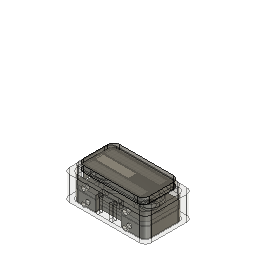
Tactile Sensor MK2 v15 (Autodesk Fusion 360 design; units mm, degrees)
Autodesk Fusion 360 part; units mm, degrees
(part 1 of 2)
sketch "Sketch1" plane through (0, 0, 0) normal (0, 0, 1) x (1, 0, 0)
  line L0 (16.51, 9.525) -> (-16.51, 9.525)
  line L1 (-16.51, 9.525) -> (-16.51, -9.525)
  line L2 (-16.51, -9.525) -> (16.51, -9.525)
  line L3 (16.51, -9.525) -> (16.51, 9.525)
  line L4 (16.51, 9.525) -> (-16.51, -9.525) construction
  line L5 (-16.51, 9.525) -> (16.51, -9.525) construction
  dimension "d1" = 33.02
  dimension "d2" = 19.05
  constraint horizontal L0
  constraint perpendicular L0 L1
  constraint parallel L0 L2
  constraint parallel L1 L3
  constraint coincident L4 origin
  constraint coincident L5 origin
  measures "d1" distance of L0.start L0.end
  measures "d2" distance of L0.start L2.end
extrude "Extrude1" add sketch "Sketch1" along normal mid plane 12.7 makes body 1
sketch "Sketch3" plane through (0, 0, 0) normal (0, 1, 0) x (1, 0, 0) in component "1"
  line L0 (21, -3) -> (-21, -3)
  line L1 (-21, -3) -> (-21, 3)
  line L2 (-21, 3) -> (21, 3)
  line L3 (21, 3) -> (21, -3)
  line L4 (21, -3) -> (-21, 3) construction
  line L5 (-21, -3) -> (21, 3) construction
  dimension "d5" = 6
  dimension "d7" = 42
  constraint horizontal L0
  constraint perpendicular L0 L1
  constraint parallel L0 L2
  constraint parallel L1 L3
  constraint coincident L4 origin
  constraint coincident L5 origin
  measures "d5" distance of L0.end L1.end
  measures "d7" distance of L1.end L2.end
extrude "Extrude1'" add sketch "Sketch3" along normal mid plane 22 separate body makes body 2 in component "1"
sketch "Sketch1 (2)" plane through (0, 0, 0) normal (0, 0, 1) x (1, 0, 0) in component "49E Hall Sensor LM393"
  line L0 (13.7, 7.8) -> (-13.7, 7.8)
  line L1 (-13.7, 7.8) -> (-13.7, -7.8)
  line L2 (-13.7, -7.8) -> (13.7, -7.8)
  line L3 (13.7, -7.8) -> (13.7, 7.8)
  line L4 (13.7, 7.8) -> (-13.7, -7.8) construction
  line L5 (-13.7, 7.8) -> (13.7, -7.8) construction
  dimension "d279" = 27.4
  dimension "d280" = 15.6
  constraint horizontal L0
  constraint perpendicular L0 L1
  constraint parallel L0 L2
  constraint parallel L1 L3
  constraint coincident L4 origin
  constraint coincident L5 origin
  measures "d279" distance of L0.start L0.end
  measures "d280" distance of L0.start L2.end
extrude "Extrude1''" add sketch "Sketch1 (2)" along normal blind 1.55 separate body makes body 3 in component "49E Hall Sensor LM393"
sketch "Sketch2" plane through (0, 0, 1.55) normal (0, 0, 1) x (-1, 0, 0) in component "49E Hall Sensor LM393"
  line L0 (-18.2, -2) -> (-14.4, -2)
  line L1 (-14.4, -2) -> (-14.4, 2)
  line L2 (-14.4, 2) -> (-18.2, 2)
  line L3 (-18.2, 2) -> (-18.2, -2)
  line L4 (-18.2, -2) -> (-14.4, 2) construction
  line L5 (-14.4, -2) -> (-18.2, 2) construction
  line L6 (-13.7, 7.8) -> (-13.7, -7.8)
  line L7 (-13.7, -7.8) -> (13.7, -7.8)
  line L8 (13.7, -7.8) -> (13.7, 7.8)
  line L9 (13.7, 7.8) -> (-13.7, 7.8)
  line L10 (0, 0) -> (-16.3, 0) construction
  line L11 (-13.7, -1.2) -> (-14.4, -1.2)
  line L12 (-14.4, -1.2) -> (-14.4, 1.2)
  line L13 (-14.4, 1.2) -> (-13.7, 1.2)
  line L14 (-13.7, 1.2) -> (-13.7, -1.2)
  line L15 (-13.7, -1.2) -> (-14.4, 1.2) construction
  line L16 (-14.4, -1.2) -> (-13.7, 1.2) construction
  point P0 (-16.3, 0)
  point P1 (-14.05, 0)
  dimension "d16" = 4
  dimension "d281" = 2.4
  dimension "d282" = 4.5
  dimension "d283" = 0.7
  constraint horizontal L0
  constraint perpendicular L0 L1
  constraint parallel L0 L2
  constraint parallel L1 L3
  constraint coincident L4 P0
  constraint coincident L5 P0
  constraint coincident L10.start origin
  constraint perpendicular L3 L10
  constraint coincident P0 L10.end
  constraint horizontal L11
  constraint perpendicular L11 L12
  constraint parallel L11 L13
  constraint parallel L12 L14
  constraint coincident L6 L11.start
  constraint coincident L15 P1
  constraint coincident L16 P1
  constraint coincident L10 P1
  constraint coincident L1 L11.end
  measures "d16" distance of L0.start L2.end
  measures "d281" distance of L11.start L13.end
  measures "d282" distance of L3 L6
  measures "d283" distance of L1 L6
extrude "Extrude2" add sketch "Sketch2" along normal blind 1 separate body contours L0 L1 L2 L3 L12 makes body 4 in component "49E Hall Sensor LM393"
extrude "Extrude4" add sketch "Sketch2" against normal blind 0.5 contours L0 L1 L2 L3 L12 | L1 L6 L11 L12 L13 L14 bodies 3 4 in component "49E Hall Sensor LM393"
sketch "Sketch7" plane through (0, 0, 3) normal (0, 0, 1) x (-1, 0, 0) in component "1"
  line L0 (21, -9) -> (-19, -9)
  line L1 (-19, -9) -> (-19, 9)
  line L2 (-19, 9) -> (21, 9)
  line L3 (21, 9) -> (21, -9)
  line L4 (21, -9) -> (-19, 9) construction
  line L5 (-19, -9) -> (21, 9) construction
  line L6 (-21, 11) -> (-21, -11)
  line L7 (-21, -11) -> (21, -11)
  line L8 (21, -11) -> (21, 11)
  line L9 (21, 11) -> (-21, 11)
  line L10 (0, 0) -> (21, 0) construction
  line L11 (19, -9) -> (19, 9)
  point P0 (1, 0)
  dimension "d301" = 2
  dimension "d302" = 2
  dimension "d455" = 2
  constraint horizontal L0
  constraint perpendicular L0 L1
  constraint parallel L0 L2
  constraint parallel L1 L3
  constraint coincident L4 P0
  constraint coincident L5 P0
  constraint coincident L10.start origin
  constraint midpoint L8 L10.end
  constraint coincident P0 L10
  constraint coincident L0.start L8
  constraint coincident L0 L11.start
  constraint coincident L2 L11.end
  constraint perpendicular L2 L11
  measures "d301" distance of L0 L7
  measures "d302" distance of L1 L6
  measures "d455" distance of L3 L11
extrude "Extrude12" cut sketch "Sketch7" against normal blind 4 contours L0 L1 L2 L11 bodies 2 in component "1"
sketch "Sketch9" plane through (0, 0, -1) normal (0, 0, 1) x (-1, 0, 0) in component "1"
  line L0 (21, -9.9472) -> (21, 9.9472)
  line L1 (-17, 9.9472) -> (-17, -9.9472) construction
  line L2 (-8, -5.8) -> (-8, 5.8) construction
  circle A0 centre (-8, -5.8) radius 0.8
  circle A1 centre (-8, 5.8) radius 0.8
  line L3 (19, 9) -> (-19, 9)
  line L4 (-19, 9) -> (-19, -9)
  line L5 (-1.5368, 0) -> (0, 0)
  line L6 (0, 0) -> (19, 0) construction
  line L7 (19, -9) -> (19, 9)
  point P0 (-1.5368, 0)
  point P1 (-8, 0)
  dimension "d53" = 11.6
  dimension "d305" = 11
  dimension "d306" = 1.6
  constraint coincident L2.start A0.centre
  constraint coincident L2.end A1.centre
  constraint equal A0 A1
  constraint coincident P0 L5.start
  constraint coincident L5.end L6.start
  constraint horizontal L5
  constraint midpoint L2 P1
  constraint coincident L6 P1
  constraint vertical L2
  constraint midpoint L6.end L7
  measures "d53" distance of L2.start L2.end
  measures "d305" distance of L2 L4
  measures "d306" diameter of A0
extrude "Extrude7" add sketch "Sketch9" along normal blind 4 bodies 2 in component "1"
sketch "Sketch15" plane through (0, 0, 3) normal (0, 0, 1) x (-1, 0, 0) in component "1"
  line L0 (-21, -11) -> (21, -11)
  line L1 (19, -9) -> (-19, -9)
  line L2 (-19, -9) -> (-19, 9)
  line L3 (-19, 9) -> (19, 9)
  line L4 (21, -11) -> (21, 11)
  line L5 (21, 11) -> (-21, 11)
  line L6 (-21, 11) -> (-21, -11)
  circle A0 centre (-8.5, 0) radius 11.5
  line L7 (0, 0) -> (-21, 0) construction
  line L8 (19, 9) -> (19, -9)
  dimension "d407" = 23
  dimension "d408" = 12.5
  constraint coincident L7.start origin
  constraint midpoint L6 L7.end
  constraint coincident A0.centre L7
  measures "d407" diameter of A0
  measures "d408" distance of L6 A0.centre
sketch "Sketch13" plane through (0, 0, -3) normal (0, 0, -1) x (1, 0, 0) in component "1"
  line L0 (21, -11) -> (21, 11)
  line L1 (21, 11) -> (-21, 11)
  line L2 (-21, 11) -> (-21, -11)
  line L3 (-21, -11) -> (21, -11)
  line L4 (-21, 6) -> (-17, 6)
  line L5 (-17, 6) -> (-17, -6)
  line L6 (-17, -6) -> (-21, -6)
  line L7 (-21, -6) -> (-21, 6)
  line L8 (-21, 6) -> (-17, -6) construction
  line L9 (-17, 6) -> (-21, -6) construction
  line L10 (0, 0) -> (-21, 0)
  point P0 (-19, 0)
  dimension "d309" = 4
  dimension "d310" = 12
  constraint horizontal L4
  constraint perpendicular L4 L5
  constraint parallel L4 L6
  constraint parallel L5 L7
  constraint coincident L2 L4.start
  constraint coincident L8 P0
  constraint coincident L9 P0
  constraint coincident L10.start origin
  constraint midpoint L7 L10.end
  constraint horizontal L10
  measures "d309" distance of L4.start L4.end
  measures "d310" distance of L4.end L5.end
sketch "Sketch3 (2)" plane through (0, 0, 0) normal (0, 1, 0) x (1, 0, 0) in component "cap 1"
  line L0 (21, -0.75) -> (-21, -0.75)
  line L1 (-21, -0.75) -> (-21, 0.75)
  line L2 (-21, 0.75) -> (21, 0.75)
  line L3 (21, 0.75) -> (21, -0.75)
  line L4 (21, -0.75) -> (-21, 0.75) construction
  line L5 (-21, -0.75) -> (21, 0.75) construction
  dimension "d5_1" = 1.5
  dimension "d7_1" = 42
  constraint horizontal L0
  constraint perpendicular L0 L1
  constraint parallel L0 L2
  constraint parallel L1 L3
  constraint coincident L4 origin
  constraint coincident L5 origin
  measures "d5_1" distance of L0.end L1.end
  measures "d7_1" distance of L1.end L2.end
extrude "Extrude1'''" add sketch "Sketch3 (2)" along normal mid plane 25 separate body makes body 5 in component "cap 1"
sketch "Sketch20" plane through (0, 0, -0.75) normal (0, 0, -1) x (1, 0, 0) in component "cap 1"
  line L0 (-21, 12.5) -> (-21, -12.5)
  line L1 (-21, -12.5) -> (21, -12.5)
  line L2 (21, -12.5) -> (21, 12.5)
  line L3 (21, 12.5) -> (-21, 12.5)
  line L4 (18.8, 10.3) -> (-21, 10.3)
  line L5 (-21, 10.3) -> (-21, -10.3)
  line L6 (-21, -10.3) -> (18.8, -10.3)
  line L7 (18.8, -10.3) -> (18.8, 10.3)
  line L8 (18.8, 10.3) -> (-21, -10.3) construction
  line L9 (-21, 10.3) -> (18.8, -10.3) construction
  line L10 (21, 0) -> (-21, 0) construction
  point P0 (-1.1, 0)
  dimension "d316" = 2.2
  dimension "d317" = 2.2
  constraint horizontal L4
  constraint perpendicular L4 L5
  constraint parallel L4 L6
  constraint parallel L5 L7
  constraint coincident L8 P0
  constraint coincident L9 P0
  constraint midpoint L2 L10.start
  constraint midpoint L0 L10.end
  constraint coincident P0 L10
  constraint coincident L0 L4.end
  measures "d316" distance of L3 L4
  measures "d317" distance of L2 L7
extrude "Extrude23" add sketch "Sketch20" along normal blind 1.5 contours L0 L4 L5 L6 L7 bodies 5 in component "cap 1"
fillet "Fillet2" radius 3.5 2 edges at (21, -12.5, 0) (21, 12.5, 0) on bodies 5 in component "cap 1"
fillet "Fillet2" radius 3.5 2 edges at (18.8, -10.3, -1.5) (18.8, 10.3, -1.5) on bodies 5 in component "cap 1"
sketch "Sketch18" plane through (0, 0, 0.75) normal (0, 0, 1) x (1, 0, 0) in component "cap 1"
  line L0 (21, -9) -> (21, 9)
  arc A0 (21, 9) -> (17.5, 12.5) centre (17.5, 9) ccw
  line L1 (17.5, 12.5) -> (-21, 12.5)
  line L2 (-21, 12.5) -> (-21, -12.5)
  line L3 (-21, -12.5) -> (17.5, -12.5)
  arc A1 (17.5, -12.5) -> (21, -9) centre (17.5, -9) ccw
  line L4 (21, -9) -> (21, 9)
  line L5 (0, 0) -> (21, 0)
  circle A2 centre (8.5, 0) radius 12.5
  constraint coincident L5.start origin
  constraint midpoint L4 L5.end
  constraint coincident L5 A2.centre
  constraint tangent L1 A2
  constraint tangent L0 A2
sketch "Sketch21" plane through (0, 0, 0.75) normal (0, 0, 1) x (-1, 0, 0) in component "cap 1"
  circle A0 centre (-8.5, 0) radius 9.5
  arc A1 (-18.8, -6.8) -> (-15.3, -10.3) centre (-15.3, -6.8) ccw
  line L0 (-18.8, -6.8) -> (-18.8, 6.8)
  arc A2 (-15.3, 10.3) -> (-18.8, 6.8) centre (-15.3, 6.8) ccw
  line L1 (-15.3, 10.3) -> (21, 10.3)
  line L2 (21, 10.3) -> (21, -10.3)
  line L3 (21, -10.3) -> (-15.3, -10.3)
  line L4 (1.8, -10.3) -> (1.8, 10.3)
  arc A3 (-21, -9) -> (-17.5, -12.5) centre (-17.5, -9) ccw
  line L5 (-17.5, -12.5) -> (21, -12.5)
  line L6 (21, -12.5) -> (21, 12.5)
  line L7 (21, 12.5) -> (-17.5, 12.5)
  arc A4 (-17.5, 12.5) -> (-21, 9) centre (-17.5, 9) ccw
  line L8 (-21, 9) -> (-21, -9)
  line L9 (0, 0) -> (-18.8, 0) construction
  dimension "d400" = 19
  dimension "d401" = 20.6
  dimension "d406" = 12.5
  constraint coincident L3 L4.start
  constraint coincident L1 L4.end
  constraint perpendicular L1 L4
  constraint coincident L9.start origin
  constraint midpoint L0 L9.end
  constraint coincident A0.centre L9
  measures "d400" diameter of A0
  measures "d401" distance of L0 L4
  measures "d406" distance of A0.centre L8
extrude "Extrude26" cut sketch "Sketch21" against normal blind 3.1 contours A0 bodies 5 in component "cap 1"
sketch "Sketch16" plane through (0, 0, 0.75) normal (0, 0, 1) x (-1, 0, 0) in component "cap 1"
  line L0 (0, 0) -> (21, 0) construction
  line L1 (-17.5, -12.5) -> (21, -12.5)
  line L2 (21, -12.5) -> (21, 12.5)
  line L3 (21, 12.5) -> (-17.5, 12.5)
  arc A0 (-21, -9) -> (-17.5, -12.5) centre (-17.5, -9) ccw
  arc A1 (-17.5, 12.5) -> (-21, 9) centre (-17.5, 9) ccw
  line L4 (-21, 9) -> (-21, -9)
  circle A2 centre (-8.5, 0) radius 9.5
  line L5 (5, -5) -> (8, -5)
  line L6 (8, -5) -> (8, 5)
  line L7 (8, 5) -> (5, 5)
  line L8 (5, 5) -> (5, -5)
  line L9 (5, -5) -> (8, 5) construction
  line L10 (8, -5) -> (5, 5) construction
  line L11 (11, -3) -> (14, -3)
  line L12 (14, -3) -> (14, 3)
  line L13 (14, 3) -> (11, 3)
  line L14 (11, 3) -> (11, -3)
  line L15 (11, -3) -> (14, 3) construction
  line L16 (14, -3) -> (11, 3) construction
  point P0 (6.5, 0)
  point P1 (12.5, 0)
  dimension "d413" = 3
  dimension "d414" = 10
  dimension "d415" = 15
  dimension "d416" = 21
  dimension "d417" = 3
  dimension "d418" = 6
  constraint coincident L0.start origin
  constraint midpoint L0.end L2
  constraint horizontal L5
  constraint perpendicular L5 L6
  constraint parallel L5 L7
  constraint parallel L6 L8
  constraint coincident L9 P0
  constraint coincident L10 P0
  constraint coincident L0 P0
  constraint horizontal L11
  constraint perpendicular L11 L12
  constraint parallel L11 L13
  constraint parallel L12 L14
  constraint coincident L15 P1
  constraint coincident L16 P1
  constraint coincident L0 P1
  measures "d413" distance of L5.start L5.end
  measures "d414" distance of L5.start L7.end
  measures "d415" distance of A2.centre P0
  measures "d416" distance of A2.centre P1
  measures "d417" distance of L11.start L11.end
  measures "d418" distance of L11.end L12.end
extrude "Extrude16" cut sketch "Sketch16" against normal blind 3.5 contours L5 L6 L7 L8 | L11 L12 L13 L14 bodies 5 in component "cap 1"
sketch "Sketch1 (3)" plane through (0, 0, 0) normal (0, 0, 1) x (1, 0, 0) in component "FSR"
  circle A0 centre (0, 0) radius 9.25
  line L0 (-8.4107, 3.85) -> (-47.4107, 3.85)
  line L1 (-47.4107, 3.85) -> (-47.4107, -3.85)
  line L2 (-47.4107, -3.85) -> (-8.4107, -3.85)
  line L3 (-8.4107, -3.85) -> (-8.4107, 3.85)
  line L4 (-8.4107, 3.85) -> (-47.4107, -3.85) construction
  line L5 (-47.4107, 3.85) -> (-8.4107, -3.85) construction
  line L6 (0, 0) -> (-43.0818, 0) construction
  point P0 (-27.9107, 0)
  point P1 (-30.0207, -4.2733)
  dimension "d244" = 18.5
  dimension "d246" = 7.7
  dimension "d247" = 39
  constraint coincident A0.centre L6.start
  constraint horizontal L0
  constraint perpendicular L0 L1
  constraint parallel L0 L2
  constraint parallel L1 L3
  constraint coincident A0 L0.start
  constraint coincident L4 P0
  constraint coincident L5 P0
  constraint coincident P0 L6
  constraint horizontal L6
  measures "d244" diameter of A0
  measures "d246" distance of L0.end L1.end
  measures "d247" distance of L1.end L2.end
extrude "Extrude1''''" add sketch "Sketch1 (3)" along normal blind 0.06 separate body makes body 6 in component "FSR"
sketch "Sketch1 (4)" plane through (0, 0, 0) normal (0, 0, -1) x (1, 0, 0) in component "termistor"
  line L0 (-2.5, 2.5) -> (18, 2.5)
  line L1 (18, 2.5) -> (18, -2.5)
  line L2 (18, -2.5) -> (-2.5, -2.5)
  line L3 (-2.5, -2.5) -> (-2.5, 2.5)
  line L4 (-2.5, 2.5) -> (18, -2.5) construction
  line L5 (18, 2.5) -> (-2.5, -2.5) construction
  line L6 (0, 0) -> (7.75, 0) construction
  line L7 (-8.4107, 3.85) -> (-47.4107, 3.85)
  line L8 (-47.4107, 3.85) -> (-47.4107, -3.85)
  line L9 (-47.4107, -3.85) -> (-8.4107, -3.85)
  arc A0 (-8.4107, -3.85) -> (-8.4107, 3.85) centre (0, 0) ccw
  point P0 (7.75, 0)
  dimension "d160" = 5
  constraint horizontal L0
  constraint perpendicular L0 L1
  constraint parallel L0 L2
  constraint parallel L1 L3
  constraint coincident L4 P0
  constraint coincident L5 P0
  constraint coincident L6.start A0.centre
  constraint horizontal L6
  constraint coincident P0 L6.end
  measures "d160" distance of L0.start L2.end
sketch "Sketch3 (3)" plane through (0, 0, 1.55) normal (0, 0, 1) x (-1, 0, 0) in component "49E Hall Sensor LM393"
  line L0 (-13.7, 7.8) -> (-13.7, 1.2)
  line L1 (-13.7, 1.2) -> (-14.4, 1.2)
  line L2 (-14.4, 1.2) -> (-14.4, -1.2)
  line L3 (-14.4, -1.2) -> (-13.7, -1.2)
  line L4 (-13.7, -1.2) -> (-13.7, -7.8)
  line L5 (-13.7, -7.8) -> (13.7, -7.8)
  line L6 (13.7, -7.8) -> (13.7, 7.8)
  line L7 (13.7, 7.8) -> (-13.7, 7.8)
  line L8 (-11.7, -7.8) -> (-11.7, 7.8)
  line L9 (0, 0) -> (-11.7, 0)
  point P0 (-11.7, -5.8)
  point P1 (-11.7, 5.8)
  dimension "d286" = 11.6
  dimension "d287" = 5.8
  dimension "d288" = 2
  constraint coincident L5 L8.start
  constraint coincident L7 L8.end
  constraint perpendicular L7 L8
  constraint coincident L8 P0
  constraint coincident L8 P1
  constraint coincident L9.start origin
  constraint midpoint L8 L9.end
  measures "d286" distance of P0 P1
  measures "d287" distance of P1 L9
  measures "d288" distance of L0 L8
hole "Hole2" at (11.7, 5.8, 1.55) at (11.7, -5.8, 1.55) direction (0, 0, -1) diameter 2 depth 2000 tip angle 118 bodies 3 in component "49E Hall Sensor LM393"
sketch "Sketch4" plane through (0, 0, 1.55) normal (0, 0, 1) x (-1, 0, 0) in component "49E Hall Sensor LM393"
  circle A0 centre (-11.7, -5.8) radius 1
  circle A1 centre (-11.7, 5.8) radius 1
  line L0 (-13.7, 7.8) -> (-13.7, 1.2)
  line L1 (-13.7, 1.2) -> (-14.4, 1.2)
  line L2 (-14.4, 1.2) -> (-14.4, -1.2)
  line L3 (-14.4, -1.2) -> (-13.7, -1.2)
  line L4 (-13.7, -1.2) -> (-13.7, -7.8)
  line L5 (-13.7, -7.8) -> (13.7, -7.8)
  line L6 (13.7, -7.8) -> (13.7, 7.8)
  line L7 (13.7, 7.8) -> (-13.7, 7.8)
  line L8 (0, 0) -> (13.7, 0)
  line L9 (11.2, -5.5) -> (16.2, -5.5)
  line L10 (16.2, -5.5) -> (16.2, 5.5)
  line L11 (16.2, 5.5) -> (11.2, 5.5)
  line L12 (11.2, 5.5) -> (11.2, -5.5)
  line L13 (11.2, -5.5) -> (16.2, 5.5) construction
  line L14 (16.2, -5.5) -> (11.2, 5.5) construction
  point P0 (13.7, 0)
  dimension "d292" = 11
  dimension "d293" = 5
  constraint coincident L8.start origin
  constraint midpoint L6 P0
  constraint horizontal L9
  constraint perpendicular L9 L10
  constraint parallel L9 L11
  constraint parallel L10 L12
  constraint coincident L13 P0
  constraint coincident L14 P0
  constraint coincident P0 L8.end
  measures "d292" distance of L9.end L10.end
  measures "d293" distance of L9.start L9.end
extrude "Extrude5" add sketch "Sketch4" along normal blind 3 contours L6 L9 L10 L11 | L6 L8 L11 L12 | L6 L8 L9 L12 bodies 3 in component "49E Hall Sensor LM393"
extrude "Extrude1'''''" add sketch "Sketch1 (4)" along normal blind 0.2 separate body contours L0 L2 L3 A0 | L0 L1 L2 A0 makes body 7 in component "termistor"
sketch "Sketch2 (2)" plane through (0, 0, 0) normal (0, 0, 1) x (-1, 0, 0) in component "termistor"
  line L0 (-18, 2.5) -> (-18, -2.5)
  line L1 (-18, -2.5) -> (2.5, -2.5)
  line L2 (2.5, -2.5) -> (2.5, 2.5)
  line L3 (2.5, 2.5) -> (-18, 2.5)
  line L4 (-18, -2.5) -> (-17.8, -2.5)
  line L5 (-17.8, -2.5) -> (-17.8, 2.5)
  line L6 (-17.8, 2.5) -> (-18, 2.5)
  line L7 (-18, 2.5) -> (-18, -2.5)
  line L8 (-18, -2.5) -> (-17.8, 2.5) construction
  line L9 (-17.8, -2.5) -> (-18, 2.5) construction
  line L10 (-18, -0.9562) -> (-17.8, -0.9562)
  line L11 (-17.8, -0.9562) -> (-17.8, 0.9562)
  line L12 (-17.8, 0.9562) -> (-18, 0.9562)
  line L13 (-18, 0.9562) -> (-18, -0.9562)
  line L14 (-18, -0.9562) -> (-17.8, 0.9562) construction
  line L15 (-17.8, -0.9562) -> (-18, 0.9562) construction
  point P0 (-17.9, 0)
  point P1 (-17.9, 0)
  dimension "d163" = 0.2
  constraint horizontal L4
  constraint perpendicular L4 L5
  constraint parallel L4 L6
  constraint parallel L5 L7
  constraint coincident L0.end L1.start
  constraint coincident L8 P1
  constraint coincident L9 P1
  constraint coincident L0.start L3.end
  constraint horizontal L10
  constraint perpendicular L10 L11
  constraint parallel L10 L12
  constraint parallel L11 L13
  constraint coincident L7 L10.start
  constraint coincident L14 P1
  constraint coincident L15 P1
  constraint coincident P1 P0
  measures "d163" distance of L5.end L0.start
extrude "Extrude2'" add sketch "Sketch2 (2)" along normal blind 7 contours L0 L3 L5 L6 L7 L12 | L0 L1 L4 L5 L7 L10 bodies 7 in component "termistor"
sketch "Sketch1 (5)" plane through (0, 0, 0) normal (0, 0, 1) x (1, 0, 0) in component "Foam"
  circle A0 centre (0, 0) radius 9.375
  dimension "d248" = 18.75
  constraint coincident A0.centre origin
  measures "d248" diameter of A0
extrude "Extrude1''''''" add sketch "Sketch1 (5)" along normal mid plane 7 separate body makes body 8 in component "Foam"
sketch "Sketch1 (6)" plane through (0, 0, 0) normal (0, 0, 1) x (1, 0, 0) in component "FSR Load plate (1)"
  circle A0 centre (0, 0) radius 11
  circle A1 centre (0, 0) radius 9
  circle A2 centre (0, 0) radius 2.65
  dimension "d257_1" = 22
  dimension "d258_1" = 18
  dimension "d388" = 5.3
  constraint coincident A0.centre A1.centre
  constraint concentric A0 A1
  measures "d257_1" diameter of A0
  measures "d258_1" diameter of A1
  measures "d388" diameter of A2
extrude "Extrude1'''''''" add sketch "Sketch1 (6)" along normal blind 6 separate body contours A1 | A2 makes body 9 in component "FSR Load plate (1)"
extrude "Extrude2''" add sketch "Sketch1 (6)" along normal blind 1 contours A0 | A1 bodies 9 in component "FSR Load plate (1)"
sketch "Sketch14" plane through (0, 0, -1) normal (0, 0, 1) x (-1, 0, 0) in component "1"
  line L0 (-19, 9) -> (-19, -9)
  line L1 (-21, 11) -> (-21, -11)
  line L2 (-21, 11) -> (21, 11)
  line L3 (21, -11) -> (-21, -11)
  circle A0 centre (-9, 0) radius 5.85 construction
  line L4 (0, 0) -> (-19, 0) construction
  circle A1 centre (-9, 0) radius 5.45
  circle A2 centre (-9, 0) radius 4.1
  line L5 (-7.4277, -11.474) -> (-7.3724, 11.4476)
  circle A3 centre (-9, 0) radius 6.6 construction
  circle A4 centre (-9, 0) radius 7
  line L6 (-19, -9) -> (19, -9)
  line L7 (19, -9) -> (19, 9)
  line L8 (19, 9) -> (-19, 9)
  circle A5 centre (-8, 5.8) radius 0.8
  circle A6 centre (-8, -5.8) radius 0.8
  dimension "d372" = 11.7
  dimension "d373" = -0.4
  dimension "d374" = -1.75
  dimension "d375" = 1.6
  dimension "d376" = 13.2
  dimension "d379" = 0.4
  dimension "d399" = 12
  constraint coincident L4.start origin
  constraint midpoint L0 L4.end
  constraint concentric A0 A3
  constraint coincident A0.centre L4
  measures "d372" diameter of A0
  measures "d375" distance of A0.centre L5
  measures "d376" diameter of A3
  measures "d399" distance of L1 A0.centre
sketch "Sketch3 (4)" plane through (0, 0, 0) normal (0, 1, 0) x (1, 0, 0) in component "cap 2"
  line L0 (21, -0.75) -> (-21, -0.75)
  line L1 (-21, -0.75) -> (-21, 0.75)
  line L2 (-21, 0.75) -> (21, 0.75)
  line L3 (21, 0.75) -> (21, -0.75)
  line L4 (21, -0.75) -> (-21, 0.75) construction
  line L5 (-21, -0.75) -> (21, 0.75) construction
  dimension "d5_1_1" = 1.5
  dimension "d7_1_1" = 42
  constraint horizontal L0
  constraint perpendicular L0 L1
  constraint parallel L0 L2
  constraint parallel L1 L3
  constraint coincident L4 origin
  constraint coincident L5 origin
  measures "d5_1_1" distance of L0.end L1.end
  measures "d7_1_1" distance of L1.end L2.end
extrude "Extrude1''''''''" add sketch "Sketch3 (4)" along normal mid plane 25 separate body makes body 10 in component "cap 2"
sketch "Sketch20 (2)" plane through (0, 0, -0.75) normal (0, 0, -1) x (1, 0, 0) in component "cap 2"
  line L0 (-21, 12.5) -> (-21, -12.5)
  line L1 (-21, -12.5) -> (21, -12.5)
  line L2 (21, -12.5) -> (21, 12.5)
  line L3 (21, 12.5) -> (-21, 12.5)
  line L4 (18.8, 10.3) -> (-21, 10.3)
  line L5 (-21, 10.3) -> (-21, -10.3)
  line L6 (-21, -10.3) -> (18.8, -10.3)
  line L7 (18.8, -10.3) -> (18.8, 10.3)
  line L8 (18.8, 10.3) -> (-21, -10.3) construction
  line L9 (-21, 10.3) -> (18.8, -10.3) construction
  line L10 (21, 0) -> (-21, 0) construction
  point P0 (-1.1, 0)
  dimension "d316_1" = 2.2
  dimension "d317_1" = 2.2
  constraint horizontal L4
  constraint perpendicular L4 L5
  constraint parallel L4 L6
  constraint parallel L5 L7
  constraint coincident L8 P0
  constraint coincident L9 P0
  constraint midpoint L2 L10.start
  constraint midpoint L0 L10.end
  constraint coincident P0 L10
  constraint coincident L0 L4.end
  measures "d316_1" distance of L3 L4
  measures "d317_1" distance of L2 L7
extrude "Extrude23'" add sketch "Sketch20 (2)" along normal blind 1.5 contours L0 L4 L5 L6 L7 bodies 10 in component "cap 2"
fillet "Fillet2'" radius 3.5 2 edges at (21, -12.5, 0) (21, 12.5, 0) on bodies 10 in component "cap 2"
fillet "Fillet2'" radius 3.5 2 edges at (18.8, -10.3, -1.5) (18.8, 10.3, -1.5) on bodies 10 in component "cap 2"
sketch "Sketch18 (2)" plane through (0, 0, 0.75) normal (0, 0, 1) x (1, 0, 0) in component "cap 2"
  line L0 (21, -9) -> (21, 9)
  arc A0 (21, 9) -> (17.5, 12.5) centre (17.5, 9) ccw
  line L1 (17.5, 12.5) -> (-21, 12.5)
  line L2 (-21, 12.5) -> (-21, -12.5)
  line L3 (-21, -12.5) -> (17.5, -12.5)
  arc A1 (17.5, -12.5) -> (21, -9) centre (17.5, -9) ccw
  line L4 (21, -9) -> (21, 9)
  line L5 (0, 0) -> (21, 0)
  circle A2 centre (8.5, 0) radius 12.5
  constraint coincident L5.start origin
  constraint midpoint L4 L5.end
  constraint coincident L5 A2.centre
  constraint tangent L1 A2
  constraint tangent L0 A2
extrude "Extrude24" add sketch "Sketch18 (2)" along normal blind 1.7 contours A2 bodies 10 in component "cap 2"
sketch "Sketch21 (2)" plane through (0, 0, 2.45) normal (0, 0, 1) x (-1, 0, 0) in component "cap 2"
  circle A0 centre (-8.5, 0) radius 12.5
  circle A1 centre (-8.5, 0) radius 11
  circle A2 centre (-8.5, 0) radius 9.25
  circle A3 centre (-8.5, 0) radius 10.5
  dimension "d327_1" = -1.5
  dimension "d328_1" = 18.5
  dimension "d329_1" = 21
  constraint concentric A0 A2
  constraint concentric A2 A3
  measures "d328_1" diameter of A2
  measures "d329_1" diameter of A3
sketch "Sketch22" plane through (0, 0, -2.25) normal (0, 0, -1) x (1, 0, 0) in component "cap 2"
  arc A0 (15.3, -10.3) -> (18.8, -6.8) centre (15.3, -6.8) ccw
  line L0 (18.8, -6.8) -> (18.8, 6.8)
  arc A1 (18.8, 6.8) -> (15.3, 10.3) centre (15.3, 6.8) ccw
  line L1 (15.3, 10.3) -> (-21, 10.3)
  line L2 (-21, 10.3) -> (-21, -10.3)
  line L3 (-21, -10.3) -> (15.3, -10.3)
  line L4 (1.8, 10.3) -> (1.8, -10.3)
  dimension "d344_1" = 17
  constraint coincident L1 L4.start
  constraint coincident L3 L4.end
  constraint perpendicular L3 L4
  measures "d344_1" distance of L0 L4
sketch "Sketch1 (7)" plane through (0, 0, 0) normal (0, 0, 1) x (1, 0, 0) in component "FSR (1)"
  circle A0 centre (0, 0) radius 9.25
  line L0 (-8.4107, 3.85) -> (-47.4107, 3.85)
  line L1 (-47.4107, 3.85) -> (-47.4107, -3.85)
  line L2 (-47.4107, -3.85) -> (-8.4107, -3.85)
  line L3 (-8.4107, -3.85) -> (-8.4107, 3.85)
  line L4 (-8.4107, 3.85) -> (-47.4107, -3.85) construction
  line L5 (-47.4107, 3.85) -> (-8.4107, -3.85) construction
  line L6 (0, 0) -> (-43.0818, 0) construction
  point P0 (-27.9107, 0)
  point P1 (-30.0207, -4.2733)
  dimension "d244_1" = 18.5
  dimension "d246_1" = 7.7
  dimension "d247_1" = 39
  constraint coincident A0.centre L6.start
  constraint horizontal L0
  constraint perpendicular L0 L1
  constraint parallel L0 L2
  constraint parallel L1 L3
  constraint coincident A0 L0.start
  constraint coincident L4 P0
  constraint coincident L5 P0
  constraint coincident P0 L6
  constraint horizontal L6
  measures "d244_1" diameter of A0
  measures "d246_1" distance of L0.end L1.end
  measures "d247_1" distance of L1.end L2.end
extrude "Extrude1'''''''''" add sketch "Sketch1 (7)" along normal blind 0.06 separate body makes body 11 in component "FSR (1)"
sketch "Sketch1 (8)" plane through (0, 0, 0) normal (0, 0, -1) x (1, 0, 0) in component "termistor (1)"
  line L0 (-2.5, 2.5) -> (18, 2.5)
  line L1 (18, 2.5) -> (18, -2.5)
  line L2 (18, -2.5) -> (-2.5, -2.5)
  line L3 (-2.5, -2.5) -> (-2.5, 2.5)
  line L4 (-2.5, 2.5) -> (18, -2.5) construction
  line L5 (18, 2.5) -> (-2.5, -2.5) construction
  line L6 (0, 0) -> (7.75, 0) construction
  line L7 (-8.4107, 3.85) -> (-47.4107, 3.85)
  line L8 (-47.4107, 3.85) -> (-47.4107, -3.85)
  line L9 (-47.4107, -3.85) -> (-8.4107, -3.85)
  arc A0 (-8.4107, -3.85) -> (-8.4107, 3.85) centre (0, 0) ccw
  point P0 (7.75, 0)
  dimension "d160_1" = 5
  constraint horizontal L0
  constraint perpendicular L0 L1
  constraint parallel L0 L2
  constraint parallel L1 L3
  constraint coincident L4 P0
  constraint coincident L5 P0
  constraint coincident L6.start A0.centre
  constraint horizontal L6
  constraint coincident P0 L6.end
  measures "d160_1" distance of L0.start L2.end
extrude "Extrude1''''''''''" add sketch "Sketch1 (8)" along normal blind 0.2 separate body contours L0 L2 L3 A0 | L0 L1 L2 A0 makes body 12 in component "termistor (1)"
sketch "Sketch2 (3)" plane through (0, 0, 0) normal (0, 0, 1) x (-1, 0, 0) in component "termistor (1)"
  line L0 (-18, 2.5) -> (-18, -2.5)
  line L1 (-18, -2.5) -> (2.5, -2.5)
  line L2 (2.5, -2.5) -> (2.5, 2.5)
  line L3 (2.5, 2.5) -> (-18, 2.5)
  line L4 (-18, -2.5) -> (-17.8, -2.5)
  line L5 (-17.8, -2.5) -> (-17.8, 2.5)
  line L6 (-17.8, 2.5) -> (-18, 2.5)
  line L7 (-18, 2.5) -> (-18, -2.5)
  line L8 (-18, -2.5) -> (-17.8, 2.5) construction
  line L9 (-17.8, -2.5) -> (-18, 2.5) construction
  line L10 (-18, -0.9562) -> (-17.8, -0.9562)
  line L11 (-17.8, -0.9562) -> (-17.8, 0.9562)
  line L12 (-17.8, 0.9562) -> (-18, 0.9562)
  line L13 (-18, 0.9562) -> (-18, -0.9562)
  line L14 (-18, -0.9562) -> (-17.8, 0.9562) construction
  line L15 (-17.8, -0.9562) -> (-18, 0.9562) construction
  point P0 (-17.9, 0)
  point P1 (-17.9, 0)
  dimension "d163_1" = 0.2
  constraint horizontal L4
  constraint perpendicular L4 L5
  constraint parallel L4 L6
  constraint parallel L5 L7
  constraint coincident L0.end L1.start
  constraint coincident L8 P1
  constraint coincident L9 P1
  constraint coincident L0.start L3.end
  constraint horizontal L10
  constraint perpendicular L10 L11
  constraint parallel L10 L12
  constraint parallel L11 L13
  constraint coincident L7 L10.start
  constraint coincident L14 P1
  constraint coincident L15 P1
  constraint coincident P1 P0
  measures "d163_1" distance of L5.end L0.start
extrude "Extrude2'''" add sketch "Sketch2 (3)" along normal blind 7 contours L0 L3 L5 L6 L7 L12 | L0 L1 L4 L5 L7 L10 bodies 12 in component "termistor (1)"
sketch "Sketch1 (9)" plane through (0, 0, 0) normal (0, 0, 1) x (1, 0, 0) in component "Foam (1)"
  circle A0 centre (0, 0) radius 9.375
  dimension "d248_1" = 18.75
  constraint coincident A0.centre origin
  measures "d248_1" diameter of A0
extrude "Extrude1'''''''''''" add sketch "Sketch1 (9)" along normal mid plane 7 separate body makes body 13 in component "Foam (1)"
sketch "Sketch27" plane through (0, 0, -2.25) normal (0, 0, -1) x (1, 0, 0) in component "cap 1"
  line L0 (-18.4, -2.523) -> (-18.4, -0.673)
  line L1 (-18.4, -0.673) -> (-17.4, -0.673)
  line L2 (-17.4, -0.673) -> (-17.4, -2.523)
  line L3 (-17.4, -2.523) -> (-18.4, -2.523)
  line L4 (-17.4, 0.673) -> (-18.4, 0.673)
  line L5 (-18.4, 0.673) -> (-18.4, 2.523)
  line L6 (-18.4, 2.523) -> (-17.4, 2.523)
  line L7 (-17.4, 2.523) -> (-17.4, 0.673)
  line L8 (-18.4, -2.85) -> (-17.4, -2.85)
  line L9 (-17.4, -2.85) -> (-17.4, -8.15)
  line L10 (-17.4, -8.15) -> (-18.4, -8.15)
  line L11 (-18.4, -8.15) -> (-18.4, -2.85)
  line L12 (-18.4, 8.15) -> (-17.4, 8.15)
  line L13 (-17.4, 8.15) -> (-17.4, 2.85)
  line L14 (-17.4, 2.85) -> (-18.4, 2.85)
  line L15 (-18.4, 2.85) -> (-18.4, 8.15)
  circle A0 centre (8.5, 0) radius 9.5
  arc A1 (15.3, -10.3) -> (18.8, -6.8) centre (15.3, -6.8) ccw
  line L16 (18.8, -6.8) -> (18.8, 6.8)
  arc A2 (18.8, 6.8) -> (15.3, 10.3) centre (15.3, 6.8) ccw
  line L17 (15.3, 10.3) -> (-21, 10.3)
  line L18 (-21, 10.3) -> (-21, -10.3)
  line L19 (-21, -10.3) -> (15.3, -10.3)
  circle A3 centre (8.5, 0) radius 11.5
  circle A4 centre (8.5, 0) radius 9.5
  arc A5 (15.3, -10.3) -> (18.8, -6.8) centre (15.3, -6.8) ccw
  line L20 (18.8, -6.8) -> (18.8, 6.8)
  arc A6 (18.8, 6.8) -> (15.3, 10.3) centre (15.3, 6.8) ccw
  line L21 (15.3, 10.3) -> (-21, 10.3)
  line L22 (-21, 10.3) -> (-21, -10.3)
  line L23 (-21, -10.3) -> (15.3, -10.3)
  line L24 (-5, -5) -> (-8, -5)
  line L25 (-8, -5) -> (-8, 5)
  line L26 (-8, 5) -> (-5, 5)
  line L27 (-5, 5) -> (-5, -5)
  line L28 (-11, -3) -> (-14, -3)
  line L29 (-14, -3) -> (-14, 3)
  line L30 (-14, 3) -> (-11, 3)
  line L31 (-11, 3) -> (-11, -3)
  dimension "d403" = 23
  constraint concentric A0 A3
  measures "d403" diameter of A3
extrude "Extrude31" cut sketch "Sketch27" against normal blind 2 contours L19 A3 L23 | L16 L17 L19 A3 L20 L21 L23 | L16 A3 L20 | L17 A3 L21 bodies 5 in component "cap 1"
extrude "Extrude3" cut sketch "Sketch1 (6)" along normal blind 3 contours A2 bodies 9 in component "FSR Load plate (1)"
sketch "Sketch16 (2)" plane through (-21, 0, 0) normal (-1, 0, 0) x (0, -1, 0) in component "1"
  circle A0 centre (9.2616, 2) radius 2.5
  line L0 (-11, 2) -> (11, 2) construction
  circle A1 centre (-6, 2) radius 2.5
  line L1 (11, -3) -> (11, 3)
  line L2 (-11, -3) -> (-11, 3)
  line L3 (11, -3) -> (-11, -3)
  dimension "d419" = 5
  dimension "d429" = 5
  dimension "d430" = 5
  constraint coincident L0 A1.centre
  constraint equal A0 A1
  constraint coincident A0.centre L0
  constraint coincident L0.end L1
  constraint horizontal L0
  constraint coincident L0.start L2
  measures "d419" diameter of A1
  measures "d429" distance of A1.centre L3
  measures "d430" distance of A1.centre L2
sketch "Sketch17" plane through (0, 0, 3) normal (0, 0, 1) x (-1, 0, 0) in component "1"
  line L0 (21, 11) -> (-21, 11)
  line L1 (-21, 11) -> (-21, -11)
  line L2 (-21, -11) -> (21, -11)
  line L3 (-19, -9) -> (-19, 9)
  line L4 (19, 9) -> (19, -9)
  line L5 (19, -9) -> (-19, -9)
  line L6 (-19, 9) -> (19, 9)
  line L7 (21, -11) -> (21, 11)
  point P0 (1, -10.5)
  point P1 (1, 10.5)
sketch "Sketch17 (2)" plane through (0, 0, 0) normal (0, 0, 1) x (1, 0, 0) in component "gen 2"
  line L0 (19, 10.5) -> (-19, 10.5)
  line L1 (-19, 10.5) -> (-19, -10.5)
  line L2 (-19, -10.5) -> (19, -10.5)
  line L3 (19, -10.5) -> (19, 10.5)
  line L4 (19, 10.5) -> (-19, -10.5) construction
  line L5 (-19, 10.5) -> (19, -10.5) construction
  line L6 (-21.25, -12.75) -> (21.25, -12.75)
  line L7 (21.25, -12.75) -> (21.25, 12.75)
  line L8 (21.25, 12.75) -> (-21.25, 12.75)
  line L9 (-21.25, 12.75) -> (-21.25, -12.75)
  line L10 (-23, -14.5) -> (23, -14.5)
  line L11 (23, -14.5) -> (23, 14.5)
  line L12 (23, 14.5) -> (-23, 14.5)
  line L13 (-23, 14.5) -> (-23, -14.5)
  dimension "d1_1_1" = 38
  dimension "d2_1_1" = 21
  dimension "d3_1_1" = 2.25
  dimension "d24_1" = 4
  constraint horizontal L0
  constraint perpendicular L0 L1
  constraint parallel L0 L2
  constraint parallel L1 L3
  constraint coincident L4 origin
  constraint coincident L5 origin
  measures "d1_1_1" distance of L0.start L0.end
  measures "d2_1_1" distance of L0.start L2.end
extrude "Extrude17" add sketch "Sketch17 (2)" against normal blind 2 separate body contours L10 L11 L12 L13 makes body 14 in component "gen 2"
extrude "Extrude18" add sketch "Sketch17 (2)" along normal blind 2 contours L6 L7 L8 L9 | L10 L11 L12 L13 bodies 14 in component "gen 2"
fillet "Fillet12" radius 3.5 6 edges at (19, 10.5, 1) (21.25, 12.75, -1) (19, -10.5, 1) (21.25, -12.75, -1) (-19, -10.5, 1) (-19, 10.5, 1) on bodies 14 in component "gen 2"
sketch "Sketch3 (5)" plane through (0, 0, 0) normal (0, 1, 0) x (1, 0, 0) in component "3"
  line L0 (21, -3) -> (-21, -3)
  line L1 (-21, -3) -> (-21, 3)
  line L2 (-21, 3) -> (21, 3)
  line L3 (21, 3) -> (21, -3)
  line L4 (21, -3) -> (-21, 3) construction
  line L5 (-21, -3) -> (21, 3) construction
  dimension "d5_1_2_2" = 6
  dimension "d7_1_2_2" = 42
  constraint horizontal L0
  constraint perpendicular L0 L1
  constraint parallel L0 L2
  constraint parallel L1 L3
  constraint coincident L4 origin
  constraint coincident L5 origin
  measures "d5_1_2_2" distance of L0.end L1.end
  measures "d7_1_2_2" distance of L1.end L2.end
extrude "Extrude1''''''''''''" add sketch "Sketch3 (5)" along normal mid plane 22 separate body makes body 15 in component "3"
sketch "Sketch15 (2)" plane through (0, 0, 3) normal (0, 0, 1) x (-1, 0, 0) in component "3"
  line L0 (-21, 11) -> (-21, -11)
  line L1 (-21, -11) -> (21, -11)
  line L2 (21, -11) -> (21, 11)
  line L3 (21, 11) -> (-21, 11)
  line L4 (-19, -10.25) -> (19, -10.25)
  line L5 (19, -10.25) -> (19, 10.25)
  line L6 (19, 10.25) -> (-19, 10.25)
  line L7 (-19, 10.25) -> (-19, -10.25)
  line L8 (-19, -10.25) -> (19, 10.25) construction
  line L9 (19, -10.25) -> (-19, 10.25) construction
  dimension "d186_2_2" = 20.5
  dimension "d187_2_2" = 38
  constraint horizontal L4
  constraint perpendicular L4 L5
  constraint parallel L4 L6
  constraint parallel L5 L7
  constraint coincident L8 origin
  constraint coincident L9 origin
  measures "d186_2_2" distance of L4.start L6.end
  measures "d187_2_2" distance of L4.start L4.end
extrude "Extrude15" cut sketch "Sketch15 (2)" against normal blind 1.5 contours L4 L5 L6 L7 bodies 15 in component "3"
fillet "Fillet2''" radius 3.5 2 edges at (21, -11, 0) (21, 11, 0) on bodies 15 in component "3"
fillet "Fillet2''" radius 3.5 2 edges at (-21, 11, 0) (-21, -11, 0) on bodies 15 in component "3"
fillet "Fillet10" radius 3.5 4 edges at (19, -10.25, 2.25) (19, 10.25, 2.25) (-19, 10.25, 2.25) (-19, -10.25, 2.25) on bodies 15 in component "3"
sketch "Sketch16 (3)" plane through (0, 0, 1.5) normal (0, 0, 1) x (-1, 0, 0) in component "3"
  line L0 (0, 0) -> (-2.3841, 0)
  line L1 (-2.3841, 0) -> (-19, 0)
  line L2 (-19, -6.75) -> (-19, 6.75)
  line L3 (15, -5) -> (19, -5)
  line L4 (19, -5) -> (19, 5)
  line L5 (19, 5) -> (15, 5)
  line L6 (15, 5) -> (15, -5)
  line L7 (15, -5) -> (19, 5) construction
  line L8 (19, -5) -> (15, 5) construction
  line L9 (19, 6.75) -> (19, -6.75)
  point P0 (17, 0)
  dimension "d438" = 4
  dimension "d439" = 10
  constraint coincident L0.start origin
  constraint horizontal L0
  constraint parallel L0 L1
  constraint coincident L1.end L2
  constraint horizontal L3
  constraint perpendicular L3 L4
  constraint parallel L3 L5
  constraint parallel L4 L6
  constraint coincident L7 P0
  constraint coincident L8 P0
  constraint coincident L1 P0
  constraint coincident L3.end L9
  measures "d438" distance of L3.start L3.end
  measures "d439" distance of L3.start L5.end
extrude "Extrude18'" cut sketch "Sketch16 (3)" against normal blind 6 bodies 15 in component "3"
sketch "Sketch10" plane through (-0.1055, 1.0731, -3) normal (0, 0, -1) x (1, 0, 0) in component "3"
  line L0 (-15.3945, -9.1769) -> (15.6055, -9.1769)
  arc A0 (15.6055, -9.1769) -> (19.1055, -5.6769) centre (15.6055, -5.6769) ccw
  line L1 (19.1055, -5.6769) -> (19.1055, 7.8231)
  arc A1 (19.1055, 7.8231) -> (15.6055, 11.3231) centre (15.6055, 7.8231) ccw
  line L2 (15.6055, 11.3231) -> (-15.3945, 11.3231)
  arc A2 (-15.3945, 11.3231) -> (-18.8945, 7.8231) centre (-15.3945, 7.8231) ccw
  line L3 (-18.8945, 7.8231) -> (-18.8945, -5.6769)
  arc A3 (-18.8945, -5.6769) -> (-15.3945, -9.1769) centre (-15.3945, -5.6769) ccw
  arc A4 (17.6055, -9.9269) -> (21.1055, -6.4269) centre (17.6055, -6.4269) ccw
  line L4 (17.6055, -9.9269) -> (-17.3945, -9.9269)
  line L5 (-20.8945, -6.4269) -> (-20.8945, 8.5731)
  line L6 (-17.3945, 12.0731) -> (17.6055, 12.0731)
  arc A5 (21.1055, 8.5731) -> (17.6055, 12.0731) centre (17.6055, 8.5731) ccw
  line L7 (21.1055, 8.5731) -> (21.1055, -6.4269)
  line L8 (-20.8945, 1.0731) -> (21.1055, 1.0731)
  line L9 (-20.8945, -7.9269) -> (21.1055, -7.9269)
  line L10 (21.1055, -7.9269) -> (21.1055, 10.0731)
  line L11 (21.1055, 10.0731) -> (-20.8945, 10.0731)
  line L12 (-20.8945, 10.0731) -> (-20.8945, -7.9269)
  line L13 (-20.8945, -7.9269) -> (21.1055, 10.0731) construction
  line L14 (21.1055, -7.9269) -> (-20.8945, 10.0731) construction
  arc A6 (-17.3945, 12.0731) -> (-20.8945, 8.5731) centre (-17.3945, 8.5731) ccw
  arc A7 (-20.8945, -6.4269) -> (-17.3945, -9.9269) centre (-17.3945, -6.4269) ccw
  point P0 (0.1055, 1.0731)
  dimension "d216_2_2" = 18
  constraint midpoint L5 L8.start
  constraint midpoint L7 L8.end
  constraint horizontal L9
  constraint perpendicular L9 L10
  constraint parallel L9 L11
  constraint parallel L10 L12
  constraint coincident L5 L9.start
  constraint coincident L13 P0
  constraint coincident L14 P0
  constraint midpoint L8 P0
  measures "d216_2_2" distance of L9.start L11.end
sketch "Sketch12" plane through (0, 0, 3) normal (0, 0, 1) x (-1, 0, 0) in component "3"
  arc A0 (-21, -7.5) -> (-17.5, -11) centre (-17.5, -7.5) ccw
  line L0 (-17.5, -11) -> (17.5, -11)
  line L1 (17.5, 11) -> (-17.5, 11)
  arc A1 (-17.5, 11) -> (-21, 7.5) centre (-17.5, 7.5) ccw
  line L2 (-21, 7.5) -> (-21, -7.5)
  line L3 (17.5, 10) -> (-17.5, 10)
  arc A2 (-17.5, 10) -> (-20, 7.5) centre (-17.5, 7.5) ccw
  line L4 (-20, 7.5) -> (-20, -7.5)
  arc A3 (-20, -7.5) -> (-17.5, -10) centre (-17.5, -7.5) ccw
  line L5 (-17.5, -10) -> (17.5, -10)
  line L6 (17.5, -11) -> (17.5, 11)
  line L7 (15.5, -10.25) -> (-15.5, -10.25)
  line L8 (-19, -6.75) -> (-19, 6.75)
  line L9 (-15.5, 10.25) -> (15.5, 10.25)
  line L10 (19, 6.75) -> (19, -6.75)
  arc A4 (-19, -6.75) -> (-15.5, -10.25) centre (-15.5, -6.75) ccw
  arc A5 (-15.5, 10.25) -> (-19, 6.75) centre (-15.5, 6.75) ccw
  arc A6 (19, 6.75) -> (15.5, 10.25) centre (15.5, 6.75) ccw
  arc A7 (15.5, -10.25) -> (19, -6.75) centre (15.5, -6.75) ccw
  arc A8 (21, 7.5) -> (17.5, 11) centre (17.5, 7.5) ccw
  arc A9 (17.5, -11) -> (21, -7.5) centre (17.5, -7.5) ccw
  dimension "d98_2_2" = -1
  constraint coincident L0.end L6.start
  constraint coincident L1.start L6.end
sketch "Sketch13 (2)" plane through (-21, 0, 0) normal (-1, 0, 0) x (0, -1, 0) in component "3"
  line L0 (-7.5, -3) -> (7.5, -3)
  line L1 (7.5, 3) -> (-7.5, 3)
  line L2 (7.5, -3) -> (7.5, 3)
  line L3 (-7.5, 3) -> (-7.5, -3)
sketch "Sketch14 (2)" plane through (0, 0, 3) normal (0, 0, 1) x (1, 0, 0) in component "3"
  line L0 (-21, -12.5) -> (17.5, -12.5)
  arc A0 (17.5, -12.5) -> (21, -9) centre (17.5, -9) ccw
  line L1 (21, -9) -> (21, 9)
  arc A1 (21, 9) -> (17.5, 12.5) centre (17.5, 9) ccw
  line L2 (17.5, 12.5) -> (-21, 12.5)
  line L3 (-21, -10.1) -> (17.5, -10.1)
  arc A2 (17.5, -10.1) -> (18.6, -9) centre (17.5, -9) ccw
  line L4 (18.6, -9) -> (18.6, 9)
  arc A3 (18.6, 9) -> (17.5, 10.1) centre (17.5, 9) ccw
  line L5 (17.5, 10.1) -> (-21, 10.1)
  line L6 (-21, -11.1) -> (17.5, -11.1)
  arc A4 (17.5, -11.1) -> (19.6, -9) centre (17.5, -9) ccw
  line L7 (19.6, -9) -> (19.6, 9)
  arc A5 (19.6, 9) -> (17.5, 11.1) centre (17.5, 9) ccw
  line L8 (17.5, 11.1) -> (-21, 11.1)
  line L9 (-21, 12.5) -> (-21, -12.5)
  line L10 (18.3723, -9) -> (-21, -9)
  line L11 (-21, 9) -> (18.3723, 9)
  arc A6 (19, 7) -> (18.3723, 9) centre (15.5, 7) ccw
  line L12 (19, 7) -> (19, -7)
  arc A7 (18.3723, -9) -> (19, -7) centre (15.5, -7) ccw
  line L13 (-15.5, 10.25) -> (15.5, 10.25)
  arc A8 (19, 6.75) -> (15.5, 10.25) centre (15.5, 6.75) ccw
  line L14 (19, 6.75) -> (19, -6.75)
  arc A9 (15.5, -10.25) -> (19, -6.75) centre (15.5, -6.75) ccw
  line L15 (15.5, -10.25) -> (-15.5, -10.25)
  arc A10 (-19, -6.75) -> (-15.5, -10.25) centre (-15.5, -6.75) ccw
  line L16 (-19, -6.75) -> (-19, 6.75)
  arc A11 (-15.5, 10.25) -> (-19, 6.75) centre (-15.5, 6.75) ccw
  arc A12 (21, 7.5) -> (17.5, 11) centre (17.5, 7.5) ccw
  line L17 (17.5, 11) -> (-17.5, 11)
  line L18 (-21, 7.5) -> (-21, -7.5)
  line L19 (-17.5, -11) -> (17.5, -11)
  arc A13 (17.5, -11) -> (21, -7.5) centre (17.5, -7.5) ccw
  line L20 (21, -7.5) -> (21, 7.5)
  arc A14 (-21, -7.5) -> (-17.5, -11) centre (-17.5, -7.5) ccw
  arc A15 (-17.5, 11) -> (-21, 7.5) centre (-17.5, 7.5) ccw
  dimension "d136_2_2" = -2.4
  dimension "d137_2_2" = -1.4
  constraint coincident L2.end L9.start
  constraint coincident L0.start L9.end
sketch "Sketch3 (6)" plane through (0, 0, 0) normal (0, 1, 0) x (1, 0, 0) in component "2"
  line L0 (21, -1) -> (-21, -1)
  line L1 (-21, -1) -> (-21, 1)
  line L2 (-21, 1) -> (21, 1)
  line L3 (21, 1) -> (21, -1)
  line L4 (21, -1) -> (-21, 1) construction
  line L5 (-21, -1) -> (21, 1) construction
  dimension "d5_1_3" = 2
  dimension "d7_1_3" = 42
  constraint horizontal L0
  constraint perpendicular L0 L1
  constraint parallel L0 L2
  constraint parallel L1 L3
  constraint coincident L4 origin
  constraint coincident L5 origin
  measures "d5_1_3" distance of L0.end L1.end
  measures "d7_1_3" distance of L1.end L2.end
extrude "Extrude1'''''''''''''" add sketch "Sketch3 (6)" along normal mid plane 22 separate body makes body 16 in component "2"
fillet "Fillet11" radius 3.5 4 edges at (-21, 11, 0) (-21, -11, 0) (21, -11, 0) (21, 11, 0) on bodies 16 in component "2"
sketch "Sketch28" plane through (0, 0, 1) normal (0, 0, 1) x (-1, 0, 0) in component "2"
  arc A0 (-21, -7.5) -> (-17.5, -11) centre (-17.5, -7.5) ccw
  line L0 (-17.5, -11) -> (17.5, -11)
  arc A1 (17.5, -11) -> (21, -7.5) centre (17.5, -7.5) ccw
  line L1 (21, -7.5) -> (21, 7.5)
  arc A2 (21, 7.5) -> (17.5, 11) centre (17.5, 7.5) ccw
  line L2 (17.5, 11) -> (-17.5, 11)
  arc A3 (-17.5, 11) -> (-21, 7.5) centre (-17.5, 7.5) ccw
  line L3 (-21, 7.5) -> (-21, -7.5)
  line L4 (21, 0) -> (18.9121, 0)
  line L5 (18.9121, 0) -> (-21, 0) construction
  circle A4 centre (12.6, 0) radius 4.5
  circle A5 centre (-8, 0) radius 6.5
  circle A6 centre (12.6, 0) radius 5.5 construction
  circle A7 centre (12.6, 0) radius 6.5
  circle A8 centre (-8, 0) radius 4.5
  dimension "d472" = 8.4
  dimension "d473" = 11
  dimension "d474" = 1
  dimension "d475" = 1
  dimension "d553" = 13
  constraint midpoint L1 L4.start
  constraint perpendicular L1 L4
  constraint midpoint L3 L5.end
  constraint perpendicular L3 L5
  constraint coincident L5 A4.centre
  constraint coincident L5 A5.centre
  constraint concentric A4 A6
  constraint concentric A6 A7
  constraint concentric A5 A8
  constraint equal A4 A8
  constraint equal A5 A7
  measures "d472" distance of L4.start A4.centre
  measures "d473" diameter of A6
  measures "d474" distance of A6 A7
  measures "d475" distance of A4 A6
  measures "d553" distance of L5.end A5.centre
extrude "Extrude32" cut sketch "Sketch28" against normal blind 1.5 contours A5 | A7 bodies 16 in component "2"
sketch "Sketch20 (3)" plane through (0, 0, -1) normal (0, 0, -1) x (1, 0, 0) in component "2"
  line L0 (-21, 7.5) -> (-21, -7.5)
  line L1 (-17.5, -11) -> (17.5, -11)
  line L2 (21, -7.5) -> (21, 7.5)
  line L3 (17.5, 11) -> (-17.5, 11)
  line L4 (18.8, 8.8) -> (-21, 8.8)
  line L5 (-21, 8.8) -> (-21, -8.8)
  line L6 (-21, -8.8) -> (18.8, -8.8)
  line L7 (18.8, -8.8) -> (18.8, 8.8)
  line L8 (18.8, 8.8) -> (-21, -8.8) construction
  line L9 (-21, 8.8) -> (18.8, -8.8) construction
  line L10 (21, 0) -> (-21, 0) construction
  arc A0 (17.5, -11) -> (21, -7.5) centre (17.5, -7.5) ccw
  arc A1 (21, 7.5) -> (17.5, 11) centre (17.5, 7.5) ccw
  arc A2 (-17.5, 11) -> (-21, 7.5) centre (-17.5, 7.5) ccw
  arc A3 (-21, -7.5) -> (-17.5, -11) centre (-17.5, -7.5) ccw
  point P0 (-1.1, 0)
  dimension "d316_2" = 2.2
  dimension "d317_2" = 2.2
  constraint horizontal L4
  constraint perpendicular L4 L5
  constraint parallel L4 L6
  constraint parallel L5 L7
  constraint coincident L8 P0
  constraint coincident L9 P0
  constraint midpoint L2 L10.start
  constraint midpoint L0 L10.end
  constraint coincident P0 L10
  constraint coincident L0 L4.end
  measures "d316_2" distance of L3 L4
  measures "d317_2" distance of L2 L7
sketch "Sketch18 (3)" plane through (0, 0, 1) normal (0, 0, 1) x (1, 0, 0) in component "2"
  line L0 (21, -9) -> (21, 9)
  line L1 (0, 0) -> (21, 0)
  circle A0 centre (10, 0) radius 11
  arc A1 (21, 7.5) -> (17.5, 11) centre (17.5, 7.5) ccw
  line L2 (17.5, 11) -> (-17.5, 11)
  arc A2 (-17.5, 11) -> (-21, 7.5) centre (-17.5, 7.5) ccw
  line L3 (-21, 7.5) -> (-21, -7.5)
  arc A3 (-21, -7.5) -> (-17.5, -11) centre (-17.5, -7.5) ccw
  line L4 (-17.5, -11) -> (17.5, -11)
  arc A4 (17.5, -11) -> (21, -7.5) centre (17.5, -7.5) ccw
  line L5 (21, -7.5) -> (21, 7.5)
  circle A5 centre (8, 0) radius 6.5
  circle A6 centre (-12.6, 0) radius 6.5
  constraint coincident L1.start origin
  constraint coincident L1 A0.centre
  constraint tangent L0 A0